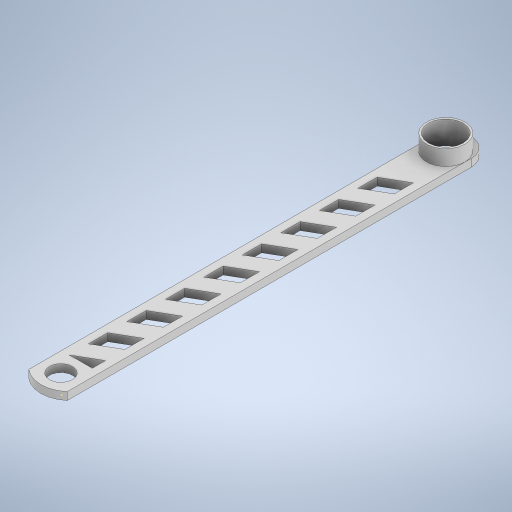
# Autodesk Inventor part: arm_v2(base-arm)
Saved by Autodesk Inventor 2024.3 (Build 283343000, 343)
## iProperties
Created: 2024-07-09
Part Number: arm_v2(base-arm)
Material: Ogólny
Document SubType Name: Modeling
Designer: User
Density: 1 g/cm^3
Appearance: Domyślna
Author: User
Autodesk Inventor part; units mm, degrees
ref_plane "YZ Plane" through (0, 0, 0) normal (1, 0, 0) x (0, 1, 0)
ref_plane "XZ Plane" through (0, 0, 0) normal (0, 1, 0) x (-1, 0, 0)
sketch "Szkic3" plane through (0, 0, 0) normal (0, 1, 0) x (-1, 0, 0)
  line L0 (0, 0) -> (10, 0)
  line L1 (10, 0) -> (10, -50)
  line L2 (10, -50) -> (0, -50)
  line L3 (0, -50) -> (0, 0)
  circle A0 centre (5, -5) radius 2.5
  arc A1 (10, -2.5) -> (0, -2.5) centre (5, -6.25) ccw
  line L4 (8, -50) -> (2, -50)
  line L5 (2, -50) -> (2, -10)
  line L6 (2, -10) -> (8, -10)
  line L7 (8, -10) -> (8, -50)
  line L8 (2, -10) -> (8, -16)
  line L9 (2, -10) -> (10.4853, -10) construction
  line L10 (8, -16) -> (8, -18)
  line L11 (8, -18) -> (2, -12)
  line L12 (2, -10) -> (2, -12)
  line L13 (8, -18) -> (8, -22)
  line L14 (2, -16) -> (8, -22)
  line L15 (8, -24) -> (2, -18)
  line L16 (8, -16) -> (8, -14)
  line L17 (8, -24) -> (8, -26)
  line L18 (2, -20) -> (8, -26)
  line L19 (8, -28) -> (2, -22)
  line L20 (8, -28) -> (8, -32)
  line L21 (2, -26) -> (8, -32)
  line L22 (8, -34) -> (2, -28)
  line L23 (8, -34) -> (8, -36)
  line L24 (2, -26) -> (8, -32)
  line L25 (8, -34) -> (2, -28)
  line L26 (8, -34) -> (8, -38)
  line L27 (2, -32) -> (8, -38)
  line L28 (8, -40) -> (2, -34)
  line L29 (8, -40) -> (8, -42)
  line L30 (2, -32) -> (8, -38)
  line L31 (8, -40) -> (2, -34)
  line L32 (8, -40) -> (8, -44)
  line L33 (2, -38) -> (8, -44)
  line L34 (8, -46) -> (2, -40)
  line L35 (8, -46) -> (8, -48)
  line L36 (2, -38) -> (8, -44)
  line L37 (8, -46) -> (2, -40)
  line L38 (8, -46) -> (8, -50)
  line L39 (8, -46) -> (8, -48)
  line L40 (8, -48) -> (2, -42)
  line L41 (2, -42) -> (2, -44)
  line L42 (2, -44) -> (8, -50)
  line L43 (7, -49) -> (2, -49)
  circle A2 centre (5, -5) radius 3.25
  dimension "d9" = 10
  dimension "d10" = 50
  dimension "d11" = 5
  dimension "d12" = 6
  dimension "d13" = 40
  dimension "d14" = 45
  dimension "d15" = 2
  dimension "d16" = 4
  dimension "d17" = 2
  dimension "d18" = 2
  dimension "d19" = 2
  dimension "d20" = 2
  dimension "d21" = 4
  dimension "d22" = 2
  dimension "d23" = 2
  dimension "d24" = 2
  dimension "d25" = 4
  dimension "d26" = 2
  dimension "d27" = 2
  dimension "d28" = 2
  dimension "d29" = 4
  dimension "d30" = 2
  dimension "d32" = 2
  dimension "d36" = 2
  dimension "d37" = 2
  dimension "d42" = 6.5
  constraints: 88 end point, 14 point on line, 13 parallel, 3 centre point, 3 horizontal, 3 perpendicular, 2 collinear, 2 point on circle, 1 coincident, 1 equal length
  measures "d9" distance of L1.end L2.end
  measures "d10" distance of L0.end L1.end
  measures "d11" diameter of A0
  measures "d12" distance of L5.end L6.end
  measures "d13" distance of L4.end L5.end
  measures "d14" angle of L8 L9
  measures "d15" distance of L8.end L10.end
  measures "d16" distance of L10.end L13.end
  measures "d17" distance of L14.end L15.start
  measures "d18" distance of L8.end L16.end
  measures "d19" distance of L15.start L17.end
  measures "d20" distance of L18.end L20.start
  measures "d21" distance of L20.start L20.end
  measures "d22" distance of L21.end L23.start
  measures "d23" distance of L23.start L23.end
  measures "d24" distance of L24.end L26.start
  measures "d25" distance of L26.start L26.end
  measures "d26" distance of L27.end L29.start
  measures "d27" distance of L29.start L29.end
  measures "d28" distance of L30.end L32.start
  measures "d29" distance of L32.start L32.end
  measures "d30" distance of L33.end L35.start
  measures "d32" distance of L36.end L38.start
  measures "d36" distance of L38.start L35.end
  measures "d37" distance of L40.end L41.end
  measures "d42" diameter of A2
extrude "Wyciągnięcie proste2" add sketch "Szkic3" against normal blind 2 contours A1 L1 L2 L7 L6 L5 L3 | L5 L43 L42 L2 | L42 L5 L40 L7 | L34 L5 L33 L7 | L28 L5 L27 L7 | L5 L21 L7 L22 | L5 L18 L7 L19 | L5 L14 L7 L15 | L5 L8 L7 L11 | A2
ref_plane "Płaszczyzna konstrukcyjna1" through (0, 0, -50) normal (0, 0, -1) x (-1, 0, 0)
mirror "Odbij1" about plane through (0, 0, -50) normal (0, 0, -1) of "Wyciągnięcie proste2"
sketch "Szkic4" plane through (0, 0, 0) normal (0, 1, 0) x (1, 0, 0)
  line L0 (-7.5, 91.0504) -> (-2.5, 91.0504)
  line L1 (-2.5, 91.0504) -> (-2.5, 98.6571)
  line L2 (-2.5, 98.6571) -> (-7.5, 98.6571)
  line L3 (-7.5, 98.6571) -> (-7.5, 91.0504)
  point P0 (0, 0)
  constraints: 8 end point, 2 parallel, 1 horizontal, 1 perpendicular
extrude "Wyciągnięcie proste3" cut sketch "Szkic4" against normal blind 2
sketch "Szkic5" plane through (0, 0, 0) normal (0, 1, 0) x (1, 0, 0)
  line L0 (-10, 2.5) -> (-10, 97.5) projected
  line L1 (-10, 97.5) -> (-10, 67.5)
  line L2 (-10, 67.5) -> (-13, 67.5)
  line L3 (-13, 67.5) -> (-13, 97.5)
  line L4 (-13, 97.5) -> (-10, 97.5)
  arc A0 (0, 97.5) -> (-10, 97.5) centre (-5, 93.75) ccw projected
  line L5 (-5, 100) -> (-5, 49.8742)
  line L6 (-5, 100) -> (45.1258, 100) construction
  line L7 (-13, 67.5) -> (-10, 62.3038)
  line L8 (-13, 67.5) -> (-7, 67.5) construction
  line L9 (-10, 62.3038) -> (-10, 67.5)
  line L10 (0, 2.5) -> (0, 97.5)
  line L11 (0, 67.5) -> (3, 67.5)
  line L12 (3, 67.5) -> (3, 97.5)
  line L13 (3, 97.5) -> (0, 97.5)
  line L14 (3, 67.5) -> (0, 62.3038)
  arc A1 (3, 97.5) -> (-13, 97.5) centre (-5, 94.4495) ccw
  point P0 (0, 0)
  dimension "d43" = 30
  dimension "d44" = 3
  dimension "d45" = 90
  dimension "d46" = 60
  constraints: 28 end point, 5 symmetric about line, 3 perpendicular, 3 point on circle, 2 equal length, 2 horizontal, 2 point on line, 1 centre point, 1 vertical
  measures "d43" distance of L0.end L1.end
  measures "d44" distance of L1.end L2.end
  measures "d45" angle of L5 L6
  measures "d46" angle of L7 L8
extrude "Wyciągnięcie proste4" add sketch "Szkic5" against normal blind 2
sketch "Szkic6" plane through (0, 0, 0) normal (0, 1, 0) x (1, 0, 0)
  line L0 (-10, 62.3038) -> (-10, 2.5) projected
  line L1 (-10, 62.3038) -> (-10, 97.356)
  line L2 (-10, 97.356) -> (0, 97.356)
  line L3 (0, 97.356) -> (0, 62.3038)
  line L4 (0, 62.3038) -> (-10, 62.3038)
  point P0 (0, 0)
  constraints: 8 end point, 3 perpendicular, 1 vertical
extrude "Wyciągnięcie proste5" cut sketch "Szkic6" against normal blind 2
sketch "Szkic7" plane through (0, 0, 0) normal (0, 1, 0) x (1, 0, 0)
  line L0 (-10, 62.3038) -> (-8, 62.3038) projected
  line L1 (-10, 62.3038) -> (-10, 67.4287)
  line L2 (-10, 62.3038) -> (-10, 97.356) projected
  line L3 (-10, 67.4287) -> (0, 67.4287)
  line L4 (0, 62.3038) -> (0, 97.356) projected
  line L5 (0, 62.3038) -> (0, 67.4287)
  line L6 (0, 62.3038) -> (-2, 62.3038) projected
  line L7 (-10, 2.5) -> (-10, 62.3038) projected
  line L8 (0, 62.3038) -> (-10, 62.3038)
  line L9 (-10, 62.3038) -> (-10, 61.2351)
  line L10 (-10, 61.2351) -> (0, 61.2351)
  line L11 (0, 61.2351) -> (0, 62.3038)
  line L12 (-10, 61.2351) -> (0, 61.2351)
  line L13 (0, 2.5) -> (0, 62.3038) projected
  line L14 (0, 61.2351) -> (0, 67.4287)
  line L15 (0, 67.4287) -> (-10, 67.4287)
  line L16 (-10, 61.2351) -> (-10, 67.4287)
  point P0 (0, 0)
  constraints: 22 end point, 5 collinear, 4 point on line, 3 perpendicular, 1 horizontal
extrude "Wyciągnięcie proste6" add sketch "Szkic7" against normal blind 2
sketch "Szkic8" plane through (0, 0, 0) normal (0, 1, 0) x (1, 0, 0)
  line L0 (-7.5, 97.356) -> (-10, 97.356) projected
  line L1 (-10, 97.356) -> (-11, 97.356)
  line L2 (-11, 97.356) -> (-11, 67.4287)
  line L3 (-11, 67.4287) -> (-10, 67.4287)
  line L4 (-10, 67.4287) -> (-10, 97.356)
  line L5 (0, 97.356) -> (1, 97.356)
  line L6 (1, 97.356) -> (1, 67.4287)
  line L7 (1, 67.4287) -> (0, 67.4287)
  line L8 (0, 67.4287) -> (0, 97.356)
  line L9 (-11, 67.4287) -> (1, 67.4287)
  line L10 (1, 67.4287) -> (1, 72.7222)
  line L11 (1, 72.7222) -> (-11, 72.7222)
  line L12 (-11, 72.7222) -> (-11, 67.4287)
  point P0 (0, 0)
  point P1 (0, 72.7222)
  point P2 (-10, 72.7222)
  dimension "d53" = 1
  dimension "d54" = 1
  constraints: 24 end point, 6 parallel, 3 horizontal, 3 perpendicular, 3 point on line
  measures "d53" distance of L3.end L2.end
  measures "d54" distance of L6.end L7.end
extrude "Wyciągnięcie proste7" cut sketch "Szkic8" against normal blind 2 contours L4 L11 L2 L1 | L8 L5 L6 L11
sketch "Szkic9" plane through (0, 0, 0) normal (0, 1, 0) x (1, 0, 0)
  line L0 (-10, 72.7222) -> (0, 72.7222)
  line L1 (0, 72.7222) -> (0, 67.3617)
  line L2 (0, 67.3617) -> (-10, 67.3617)
  line L3 (-10, 67.3617) -> (-10, 72.7222)
  point P0 (0, 0)
  constraints: 8 end point, 2 parallel, 1 horizontal, 1 perpendicular
extrude "Wyciągnięcie proste8" add sketch "Szkic9" against normal blind 2
sketch "Szkic10" plane through (0, 0, 0) normal (0, 1, 0) x (1, 0, 0)
  point P0 (0, 0)
split "Podział1" plane through (0, 0, -50) removes the side toward (0, 0, -1)
sketch "Szkic11" plane through (0, 0, 0) normal (0, 1, 0) x (1, 0, 0)
  line L0 (-10, 2.5) -> (-10, 50) projected
  line L1 (-10, 50) -> (0, 50)
  line L2 (0, 50) -> (0, 100)
  line L3 (0, 100) -> (-10, 100)
  line L4 (-10, 100) -> (-10, 50)
  line L5 (-10, 100) -> (0, 100)
  line L6 (0, 100) -> (0, 124.634)
  line L7 (0, 124.634) -> (-10, 124.634)
  line L8 (-10, 124.634) -> (-10, 100)
  line L9 (-10, 124.634) -> (-11, 124.634)
  line L10 (-11, 124.634) -> (-11, 100)
  line L11 (-11, 100) -> (-10, 100)
  line L12 (-10, 100) -> (-10, 124.634)
  line L13 (0, 124.634) -> (1, 124.634)
  line L14 (1, 124.634) -> (1, 100)
  line L15 (1, 100) -> (0, 100)
  line L16 (0, 100) -> (0, 124.634)
  line L17 (-11, 100) -> (-9, 100) construction
  line L18 (1, 100) -> (3, 100) construction
  line L19 (-11, 124.634) -> (1, 124.634)
  line L20 (1, 124.634) -> (1, 126.634)
  line L21 (1, 126.634) -> (-11, 126.634)
  line L22 (-11, 126.634) -> (-11, 124.634)
  line L23 (-11, 100) -> (-12, 100)
  line L24 (-12, 100) -> (-12, 126.634)
  line L25 (-12, 126.634) -> (-11, 126.634)
  line L26 (-11, 126.634) -> (-11, 100)
  line L27 (1, 126.634) -> (2, 126.634)
  line L28 (2, 126.634) -> (2, 100)
  line L29 (2, 100) -> (1, 100)
  line L30 (1, 100) -> (1, 126.634)
  line L31 (-12, 100) -> (-10, 96.5359)
  line L32 (-12, 100) -> (-8, 100) construction
  line L33 (2, 100) -> (0, 96.5359)
  line L34 (2, 100) -> (6, 100) construction
  line L35 (-10, 124.634) -> (-10.5, 124.634)
  line L36 (-10.5, 124.634) -> (-10.5, 100)
  line L37 (0.5, 100) -> (0.5, 124.634)
  line L38 (0.75, 100) -> (0.75, 124.634)
  line L39 (-11, 100) -> (-10.75, 100)
  line L40 (-10.75, 100) -> (-10.75, 124.634)
  point P0 (0, 0)
  dimension "d59" = 10
  dimension "d60" = 50
  dimension "d61" = 10
  dimension "d62" = 24.634
  dimension "d63" = 1
  dimension "d64" = 1
  dimension "d67" = 2
  dimension "d68" = 1
  dimension "d69" = 1
  dimension "d70" = 60
  dimension "d71" = 120
  dimension "d90" = 0.5
  dimension "d107" = 0.25
  constraints: 80 end point, 17 parallel, 11 horizontal, 11 point on line, 8 perpendicular, 2 equal length, 2 midpoint
  measures "d59" distance of L3.end L2.end
  measures "d60" distance of L2.end L1.end
  measures "d61" distance of L7.end L6.end
  measures "d62" distance of L6.end L5.end
  measures "d63" distance of L11.end L10.end
  measures "d64" distance of L14.end L15.end
  measures "d67" distance of L20.end L19.end
  measures "d68" distance of L24.end L25.end
  measures "d69" distance of L28.end L29.end
  measures "d70" angle of L31 L32
  measures "d71" angle of L33 L34
  measures "d90" distance of L7.end L35.end
  measures "d107" distance of L10.end L39.end
extrude "Wyciągnięcie proste9" add sketch "Szkic11" against normal blind 2 contours L4 L3 L2 L1 | L31 L23 L11 L4 | L2 L15 L29 L33 | L24 L25 L22 L10 L23 | L29 L14 L20 L27 L28 | L9 L22 L21 L20 L13 L7
sketch "Szkic12" plane through (0, 0, 0) normal (0, 1, 0) x (1, 0, 0)
  line L0 (-8, 51.0298) -> (-2, 51.0298)
  line L1 (-2, 51.0298) -> (-2, 96.6875)
  line L2 (-2, 96.6875) -> (-8, 96.6875)
  line L3 (-8, 96.6875) -> (-8, 51.0298)
  line L4 (-8, 51.0298) -> (-2, 54.4939)
  line L5 (-8, 51.0298) -> (-1.0718, 51.0298) construction
  line L6 (-2, 54.4939) -> (-2, 59.4939)
  line L7 (-2, 59.4939) -> (-8, 56.0298)
  line L8 (-8, 51.0298) -> (-8, 56.0298)
  line L9 (-8, 56.0298) -> (-8, 61.0298)
  line L10 (-8, 61.0298) -> (-2, 64.4939)
  line L11 (-2, 64.4939) -> (-2, 69.4939)
  line L12 (-2, 69.4939) -> (-8, 66.0298)
  line L13 (-8, 61.0298) -> (-8, 66.0298)
  line L14 (-8, 66.0298) -> (-2, 69.4939)
  line L15 (-2, 74.4939) -> (-8, 71.0298)
  line L16 (-8, 76.0298) -> (-2, 79.4939)
  line L17 (-2, 84.4939) -> (-8, 81.0298)
  line L18 (-8, 71.0298) -> (-2, 74.4939)
  line L19 (-2, 79.4939) -> (-8, 76.0298)
  line L20 (-8, 81.0298) -> (-2, 84.4939)
  line L21 (-2, 89.4939) -> (-8, 86.0298)
  line L22 (-8, 76.0298) -> (-2, 79.4939)
  line L23 (-2, 84.4939) -> (-8, 81.0298)
  line L24 (-8, 86.0298) -> (-2, 89.4939)
  line L25 (-2, 94.4939) -> (-8, 91.0298)
  point P0 (0, 0)
  dimension "d74" = 30
  dimension "d75" = 5
  dimension "d76" = 5
  dimension "d77" = 5
  dimension "d78" = 5
  dimension "d79" = 5
  dimension "d80" = 5
  dimension "d81" = 5
  dimension "d82" = 5
  dimension "d83" = 5
  dimension "d84" = 5
  dimension "d85" = 5
  dimension "d86" = 5
  constraints: 52 end point, 7 point on line, 6 parallel, 2 collinear, 2 horizontal, 1 equal length, 1 perpendicular
  measures "d74" angle of L5 L4
  measures "d75" distance of L4.end L6.end
  measures "d76" distance of L7.end L9.end
  measures "d77" distance of L10.end L11.end
  measures "d78" distance of L14.end L15.start
  measures "d79" distance of L15.end L16.start
  measures "d80" distance of L16.end L17.start
  measures "d81" distance of L18.end L19.start
  measures "d82" distance of L19.end L20.start
  measures "d83" distance of L20.end L21.start
  measures "d84" distance of L22.end L23.start
  measures "d85" distance of L23.end L24.start
  measures "d86" distance of L24.end L25.start
extrude "Wyciągnięcie proste10" cut sketch "Szkic12" against normal blind 2 contours L3 L7 L1 L4 | L3 L12 L1 L10 | L3 L16 L1 L15 | L3 L21 L1 L17 | L3 L2 L1 L25
sketch "Szkic14" plane through (0, 0, 0) normal (0, 1, 0) x (1, 0, 0)
  arc A0 (5, 2.5) -> (15, 2.5) centre (10, 6.2465) ccw
  circle A1 centre (10, 5) radius 2.5
  line L0 (5, 2.5) -> (5, 5)
  line L1 (15, 2.5) -> (15, 5)
  line L2 (5, 5) -> (10, 104.8749)
  line L3 (10, 104.8749) -> (15, 5)
  line L4 (5.1827, 8.65) -> (14.8173, 8.65)
  line L5 (6.9979, 8.65) -> (12.6647, 8.65) construction
  line L6 (5.1827, 8.65) -> (7.1827, 8.65)
  line L7 (14.8173, 8.65) -> (12.8173, 8.65)
  line L8 (12.8173, 8.65) -> (9.8313, 56.0603)
  line L9 (9.8313, 56.0603) -> (7.1827, 8.65)
  line L10 (7.2581, 10) -> (12.7322, 10)
  point P0 (0, 0)
  dimension "d91" = 10
  dimension "d92" = 5
  dimension "d93" = 100
  dimension "d103" = 2
  dimension "d104" = 2
  constraints: 22 end point, 7 point on line, 3 horizontal, 2 centre point, 2 point on circle, 2 vertical
  measures "d91" distance of L0.start L1.start
  measures "d92" diameter of A1
  measures "d93" distance of L0.end L2.end
  measures "d103" distance of L4.start L6.end
  measures "d104" distance of L4.end L7.end
extrude "Wyciągnięcie proste11" add sketch "Szkic14" against normal blind 2 contours L0 L2 L4 L3 L1 A0 | L2 L3 L4 L8 L9 | L9 L10 L8 L4
sketch "Szkic15" plane through (0, 0, 0) normal (0, 1, 0) x (1, 0, 0)
  line L0 (-8, 91.0298) -> (-8, 96.6875) projected
  line L1 (-2, 10) -> (-8, 10) projected
  line L2 (-8, 96.6875) -> (-2, 96.6875)
  line L3 (-2, 96.6875) -> (-2, 10)
  line L4 (-2, 10) -> (-8, 10)
  line L5 (-8, 10) -> (-8, 96.6875)
  point P0 (0, 0)
  constraints: 8 end point, 2 parallel, 1 horizontal, 1 perpendicular
extrude "Wyciągnięcie proste12" cut sketch "Szkic15" against normal blind 2
sketch "Szkic19" plane through (2, 0, -100) normal (1, 0, 0) x (0, 0, -1)
  line L0 (39.9881, 21.4734) -> (-120.2221, 21.4734)
  line L1 (-120.2221, 21.4734) -> (-120.2221, -34.3653)
  line L2 (-120.2221, -34.3653) -> (39.9881, -34.3653)
  line L3 (39.9881, -34.3653) -> (39.9881, 21.4734)
  point P0 (-100, 0)
  constraints: 8 end point, 2 parallel, 1 horizontal, 1 perpendicular
extrude "Wyciągnięcie proste16" cut sketch "Szkic19" along normal blind 34.5
sketch "Szkic20" plane through (0, 0, 0) normal (0, 1, 0) x (1, 0, 0)
  line L0 (-8, 10) -> (-8, 15)
  line L1 (-8, 10) -> (-8, 96.6875) projected
  line L2 (-8, 15) -> (-2, 18.4641)
  line L3 (-2, 96.6875) -> (-2, 10) projected
  line L4 (-2, 18.4641) -> (-2, 13.4641)
  line L5 (-2, 13.4641) -> (-8, 10)
  line L6 (-2, 18.4641) -> (-2, 23.4641)
  line L7 (-2, 23.4641) -> (-8, 20)
  line L8 (-8, 20) -> (-8, 15)
  line L9 (-8, 20) -> (-8, 25)
  line L10 (-8, 25) -> (-2, 28.4641)
  line L11 (-2, 28.4641) -> (-2, 23.4641)
  line L12 (-8, 30) -> (-2, 33.4641)
  line L13 (-2, 28.4641) -> (-8, 25)
  line L14 (-2, 38.4641) -> (-8, 35)
  line L15 (-8, 40) -> (-2, 43.4641)
  line L16 (-8, 45) -> (-2, 48.4641)
  line L17 (-2, 43.4641) -> (-8, 40)
  line L18 (-2, 53.4641) -> (-8, 50)
  line L19 (-8, 55) -> (-2, 58.4641)
  line L20 (-8, 60) -> (-2, 63.4641)
  line L21 (-2, 58.4641) -> (-8, 55)
  line L22 (-2, 68.4641) -> (-8, 65)
  line L23 (-8, 70) -> (-2, 73.4641)
  line L24 (-8, 75) -> (-2, 78.4641)
  line L25 (-2, 73.4641) -> (-8, 70)
  line L26 (-2, 83.4641) -> (-8, 80)
  line L27 (-8, 85) -> (-2, 88.4641)
  line L28 (-8, 85) -> (-2, 88.4641)
  line L29 (-2, 83.4641) -> (-8, 80)
  line L30 (-2, 93.4641) -> (-8, 90)
  line L31 (-8, 95) -> (-2, 98.4641)
  line L32 (-2, 93.4641) -> (-2, 96.6875)
  line L33 (-2, 96.6875) -> (-5, 96.7321)
  line L34 (-8, 95) -> (-8, 90)
  dimension "d149" = 5
  dimension "d150" = 120
  dimension "d151" = 5
  dimension "d152" = 5
  dimension "d153" = 5
  dimension "d154" = 5
  dimension "d155" = 5
  dimension "d156" = 5
  dimension "d157" = 5
  dimension "d158" = 5
  dimension "d159" = 5
  dimension "d160" = 5
  dimension "d161" = 5
  dimension "d162" = 5
  dimension "d163" = 5
  dimension "d164" = 5
  dimension "d165" = 5
  dimension "d166" = 5
  dimension "d167" = 5
  dimension "d168" = 5
  dimension "d169" = 5
  dimension "d170" = 5
  dimension "d171" = 5
  dimension "d172" = 5
  dimension "d173" = 5
  constraints: 66 end point, 13 parallel, 7 point on line, 3 collinear, 1 midpoint
  measures "d149" distance of L0.start L0.end
  measures "d150" angle of L0 L2
  measures "d151" distance of L2.end L4.end
  measures "d152" distance of L2.end L6.end
  measures "d153" distance of L7.end L9.end
  measures "d154" distance of L13.end L12.start
  measures "d155" distance of L12.end L13.start
  measures "d156" distance of L12.end L14.start
  measures "d157" distance of L14.end L15.start
  measures "d158" distance of L17.end L16.start
  measures "d159" distance of L16.end L17.start
  measures "d160" distance of L16.end L18.start
  measures "d161" distance of L18.end L19.start
  measures "d162" distance of L21.end L20.start
  measures "d163" distance of L20.end L21.start
  measures "d164" distance of L20.end L22.start
  measures "d165" distance of L22.end L23.start
  measures "d166" distance of L25.end L24.start
  measures "d167" distance of L24.end L25.start
  measures "d168" distance of L24.end L26.start
  measures "d169" distance of L26.end L27.start
  measures "d170" distance of L29.end L28.start
  measures "d171" distance of L28.end L29.start
  measures "d172" distance of L28.end L30.start
  measures "d173" distance of L30.end L31.start
extrude "Wyciągnięcie proste17" add sketch "Szkic20" against normal blind 2 contours L0 L2 L3 L5 | L1 L10 L3 L7 | L1 L14 L3 L12 | L1 L16 L3 L15 | L1 L19 L3 L18 | L1 L22 L3 L20 | L1 L24 L3 L23 | L1 L27 L3 L26 | L1 L31 L33 L3 L30
sketch "Szkic21" plane through (0, 0, 0) normal (0, 1, 0) x (1, 0, 0)
  circle A0 centre (-5, 5) radius 2.5 projected
  circle A1 centre (-5, 5) radius 2.75
  point P0 (0, 0)
  dimension "d176" = 5.5
  constraints: 1 centre point, 1 coincident
  measures "d176" diameter of A1
extrude "Wyciągnięcie proste18" cut sketch "Szkic21" against normal blind 2
sketch "Szkic22" plane through (0, 0, 0) normal (0, 1, 0) x (1, 0, 0)
  line L0 (-11, 100) -> (1, 100) projected
  line L1 (-5, 100) -> (-7, 100)
  line L2 (-7, 100) -> (-7, 98)
  line L3 (-7, 98) -> (-5, 98)
  line L4 (-5, 98) -> (-5, 100)
  line L5 (-5, 100) -> (-3, 100)
  line L6 (-3, 100) -> (-3, 98)
  line L7 (-3, 98) -> (-5, 98)
  line L8 (-5, 98) -> (-5, 100)
  circle A0 centre (-5, 4.8618) radius 4.375
  point P0 (0, 0)
  dimension "d179" = 2
  dimension "d180" = 2
  dimension "d181" = 2
  dimension "d182" = 2
  dimension "d183" = 8.75
  constraints: 16 end point, 4 parallel, 2 horizontal, 2 perpendicular, 1 centre point, 1 midpoint
  measures "d179" distance of L3.end L2.end
  measures "d180" distance of L2.end L1.end
  measures "d181" distance of L6.end L7.end
  measures "d182" distance of L5.end L6.end
  measures "d183" diameter of A0
extrude "Wyciągnięcie proste19" cut sketch "Szkic22" against normal blind 2
sketch "Szkic23" plane through (0, 0, 0) normal (0, 1, 0) x (1, 0, 0)
  arc A0 (-10, 2.5) -> (0, 2.5) centre (-5, 6.25) ccw projected
  line L0 (-10, 2.5) -> (-10, 1.5)
  line L1 (0, 2.5) -> (0, 1.5)
  arc A1 (-10, 1.5) -> (0, 1.5) centre (-5, 7.2819) ccw
  point P0 (0, 0)
  dimension "d186" = 1
  dimension "d187" = 1
  constraints: 4 end point, 2 point on circle, 2 vertical, 1 centre point
  measures "d186" distance of L0.start L0.end
  measures "d187" distance of L1.start L1.end
extrude "Wyciągnięcie proste20" add sketch "Szkic23" against normal blind 2
sketch "Szkic24" plane through (0, 0, 0) normal (0, 1, 0) x (1, 0, 0)
  circle A0 centre (-5, 4.8618) radius 4.375 projected
  circle A1 centre (-5, 4.8618) radius 3.5
  circle A2 centre (-5, 4.8618) radius 4.375
  circle A3 centre (-5, 4.8618) radius 3
  point P0 (0, 0)
  dimension "d190" = 7
  dimension "d191" = 6
  constraints: 3 centre point, 3 coincident
  measures "d190" diameter of A1
  measures "d191" diameter of A3
extrude "Wyciągnięcie proste21" add sketch "Szkic24" against normal blind 2 contours A0 | A1
sketch "Szkic25" plane through (0, 0, 0) normal (0, 1, 0) x (1, 0, 0)
  line L0 (3.7776, 94.4401) -> (-14.9005, 94.4401)
  line L1 (-14.9005, 94.4401) -> (-14.9005, 129.9076)
  line L2 (-14.9005, 129.9076) -> (3.7776, 129.9076)
  line L3 (3.7776, 129.9076) -> (3.7776, 94.4401)
  point P0 (0, 0)
  constraints: 8 end point, 2 parallel, 1 horizontal, 1 perpendicular
extrude "Wyciągnięcie proste22" cut sketch "Szkic25" against normal blind 2
sketch "Szkic26" plane through (0, 0, 0) normal (0, 1, 0) x (1, 0, 0)
  circle A0 centre (-5, 4.8618) radius 3 projected
  line L0 (-5, 4.8618) -> (-5, 104.8618)
  line L1 (-5, 4.8618) -> (95, 4.8618) construction
  circle A1 centre (-5, 104.8618) radius 4.5
  line L2 (-10, 1.5) -> (-10, 94.4401) projected
  line L3 (-10, 94.4401) -> (0, 94.4401)
  line L4 (0, 94.4401) -> (0, 111.4401)
  line L5 (0, 111.4401) -> (-10, 111.4401)
  line L6 (-10, 111.4401) -> (-10, 94.4401)
  point P0 (0, 0)
  dimension "d196" = 100
  dimension "d197" = 90
  dimension "d198" = 9
  dimension "d199" = 17
  constraints: 12 end point, 2 horizontal, 2 parallel, 2 perpendicular, 1 centre point, 1 coincident, 1 vertical
  measures "d196" distance of L0.start L0.end
  measures "d197" angle of L1 L0
  measures "d198" diameter of A1
  measures "d199" distance of L4.end L3.end
extrude "Wyciągnięcie proste23" add sketch "Szkic26" against normal blind 2 contours L6 L5 L4 L3
fillet "Zaokrąglenie1" radius 5 2 edges at (-10, -1, -111.4401) (0, -1, -111.4401)
sketch "Szkic27" plane through (0, 0, 0) normal (0, 1, 0) x (1, 0, 0)
  circle A0 centre (-5, 104.8618) radius 4.5 projected
  circle A1 centre (-5, 104.8618) radius 4.5
  circle A2 centre (-5, 104.8618) radius 5
  line L0 (0, 1.5) -> (0, 106.4401) projected
  point P0 (0, 0)
  constraints: 2 centre point, 2 coincident, 1 tangent
extrude "Wyciągnięcie proste24" add sketch "Szkic27" along normal blind 4
